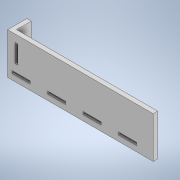
# Autodesk Inventor part: side frame left
Saved by Autodesk Inventor 2022 (Build 260153000, 153)
## iProperties
Created: 2022-04-14
Part Number: side frame left
Material: Generic
Document SubType Name: Modeling
Designer: vitalii
Density: 1 g/cm^3
Appearance: Default
Author: vitalii
Autodesk Inventor part; units mm, degrees
ref_plane "YZ Plane" through (0, 0, 0) normal (1, 0, 0) x (0, 1, 0)
ref_plane "XZ Plane" through (0, 0, 0) normal (0, 1, 0) x (-1, 0, 0)
ref_plane "XY Plane" through (0, 0, 0) normal (0, 0, 1) x (1, 0, 0)
sketch "Sketch1" plane through (0, 0, 0) normal (0, 0, 1) x (1, 0, 0)
  line L0 (-96.8016, -0.4814) -> (101.2834, -0.4814)
  line L1 (101.2834, -0.4814) -> (101.2834, -56.7314)
  line L2 (101.2834, -56.7314) -> (-96.8016, -56.7314)
  line L3 (-96.8016, -56.7314) -> (-96.8016, -0.4814)
  line L4 (-96.8016, -0.4814) -> (-90.7166, -0.4814)
  line L5 (-90.7166, -0.4814) -> (-90.7166, -56.7314)
  line L6 (-90.7166, -56.7314) -> (-96.8016, -56.7314)
  line L7 (-96.8016, -56.7314) -> (-96.8016, -0.4814)
  line L8 (-86.5466, -10.6314) -> (-82.8466, -10.6314)
  line L9 (-82.8466, -10.6314) -> (-82.8466, -35.0314)
  line L10 (-82.8466, -35.0314) -> (-86.5466, -35.0314)
  line L11 (-86.5466, -35.0314) -> (-86.5466, -10.6314)
  line L12 (-90.7166, -45.4814) -> (-65.9666, -45.4814)
  line L13 (-65.9666, -45.4814) -> (-65.9666, -48.9814)
  line L14 (-65.9666, -48.9814) -> (-90.7166, -48.9814)
  line L15 (-90.7166, -48.9814) -> (-90.7166, -45.4814)
  line L16 (-17.6566, -45.4814) -> (-17.6566, -48.9814)
  line L17 (-17.6566, -48.9814) -> (-42.4066, -48.9814)
  line L18 (-42.4066, -48.9814) -> (-42.4066, -45.4814)
  line L19 (-42.4066, -45.4814) -> (-17.6566, -45.4814)
  line L20 (30.6534, -45.4814) -> (30.6534, -48.9814)
  line L21 (30.6534, -48.9814) -> (5.9034, -48.9814)
  line L22 (5.9034, -48.9814) -> (5.9034, -45.4814)
  line L23 (5.9034, -45.4814) -> (30.6534, -45.4814)
  line L24 (78.9634, -45.4814) -> (78.9634, -48.9814)
  line L25 (78.9634, -48.9814) -> (54.2134, -48.9814)
  line L26 (54.2134, -48.9814) -> (54.2134, -45.4814)
  line L27 (54.2134, -45.4814) -> (78.9634, -45.4814)
  point P0 (0, 0)
  dimension "d0" = 198.085
  dimension "d1" = 56.25
  dimension "d2" = 0
  dimension "d3" = 0
  dimension "d4" = 0
  dimension "d5" = 6.085
  dimension "d6" = 4.17
  dimension "d7" = 10.15
  dimension "d8" = 3.7
  dimension "d9" = 24.4
  dimension "d10" = 7.75
  dimension "d11" = 0
  dimension "d12" = 24.75
  dimension "d15" = 48.31
  dimension "d20" = 3.5
  constraints: 56 end point, 6 parallel, 6 perpendicular, 5 horizontal, 1 collinear, 23 other
  measures "d0" distance of L1.end L2.end
  measures "d1" distance of L2.end L0.start
  measures "d2" distance between parallel lines of L3 L7
  measures "d3" distance between parallel lines of L2 L6
  measures "d4" distance between parallel lines of L0 L4
  measures "d5" distance between parallel lines of L3 L5
  measures "d6" distance between parallel lines of L5 L11
  measures "d7" distance between parallel lines of L0 L8
  measures "d8" distance of L8.start L8.end
  measures "d9" distance of L8.end L9.end
  measures "d10" distance between parallel lines of L2 L14
  measures "d11" distance between parallel lines of L5 L15
  measures "d12" distance of L13.end L14.end
  measures "d15" distance of L12.end L16.start
  measures "d20" distance between parallel lines of L14 L12
extrude "Extrusion1" add sketch "Sketch1" against normal blind 6.085 contours L0 L1 L2 L5 L14 L13 L12
extrude "Extrusion2" add sketch "Sketch1" against normal blind 26.125 contours L0 L5 L2 L3
sketch "Sketch2" plane through (-96.8016, -56.7314, 0) normal (-1, 0, 0) x (0, 0, 1)
  line L0 (0, 0) -> (-84, 0)
  circle A0 centre (-42, 20.75) radius 18.5
  point P0 (0, 56.7314)
  dimension "d25" = 84
  dimension "d26" = 37
  dimension "d27" = 20.75
  constraints: 2 end point, 1 centre point, 1 horizontal
  measures "d25" distance of L0.start L0.end
  measures "d26" diameter of A0
  measures "d27" distance from line of L0 A0.centre
extrude "Extrusion3" cut sketch "Sketch2" against normal blind 26.125
sketch "Sketch3" plane through (-96.8016, -56.7314, 0) normal (-1, 0, 0) x (0, 0, 1)
  line L0 (-68.8984, 11.25) -> (-12.625, 11.25)
  line L1 (-12.625, 11.25) -> (-12.625, -13.0392)
  line L2 (-12.625, -13.0392) -> (-68.8984, -13.0392)
  line L3 (-68.8984, -13.0392) -> (-68.8984, 11.25)
  line L4 (-26.125, 0) -> (-26.125, 11.2508) projected
  line L5 (0, 0) -> (-26.125, 0) projected
  point P0 (0, 56.7314)
  dimension "d30" = 13.5
  dimension "d31" = 11.25
  constraints: 8 end point, 2 parallel, 1 horizontal, 1 perpendicular
  measures "d30" distance between parallel lines of L1 L4
  measures "d31" distance between parallel lines of L5 L0
extrude "Extrusion4" cut sketch "Sketch3" against normal blind 10
body "Solid1"
